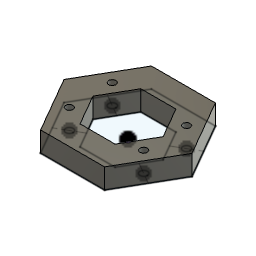
BrakeDiskSpacer (Autodesk Fusion 360 design; units mm, degrees)
Autodesk Fusion 360 part; units mm, degrees
sketch "Spacer" plane through (0, 0, 0) normal (0, 1, 0) x (1, 0, 0)
  line L0 (7.0148, 12.15) -> (-7.0148, 12.15)
  line L1 (-7.0148, 12.15) -> (-14.0296, 0)
  line L2 (-14.0296, 0) -> (-7.0148, -12.15)
  line L3 (-7.0148, -12.15) -> (7.0148, -12.15)
  line L4 (7.0148, -12.15) -> (14.0296, 0)
  line L5 (14.0296, 0) -> (7.0148, 12.15)
  line L6 (-12.7883, 22.15) -> (-25.5766, 0)
  line L7 (-25.5766, 0) -> (-12.7883, -22.15)
  line L8 (-12.7883, -22.15) -> (12.7883, -22.15)
  line L9 (12.7883, -22.15) -> (25.5766, 0)
  line L10 (25.5766, 0) -> (12.7883, 22.15)
  line L11 (12.7883, 22.15) -> (-12.7883, 22.15)
  line L12 (-19.1825, 11.075) -> (-10.5222, 6.075) construction
  line L13 (10.5222, 6.075) -> (19.1825, 11.075) construction
  line L14 (10.5222, -6.075) -> (19.1825, -11.075) construction
  line L15 (-10.5222, -6.075) -> (-19.1825, -11.075) construction
  circle A0 centre (-14.8523, 8.575) radius 1.45
  circle A1 centre (14.8523, 8.575) radius 1.45
  circle A2 centre (14.8523, -8.575) radius 1.45
  circle A3 centre (-14.8523, -8.575) radius 1.45
  dimension "d2" = 12.15
  dimension "d3" = 10
  dimension "d5" = 2.9
  dimension "d6" = 2.9
  dimension "d7" = 2.9
  dimension "d8" = 2.9
  constraint horizontal L8
  constraint horizontal L3
  constraint coincident L6 L12.start
  constraint coincident L1 L12.end
  constraint perpendicular L1 L12
  constraint midpoint L5 L13.start
  constraint midpoint L10 L13.end
  constraint midpoint L4 L14.start
  constraint coincident L9 L14.end
  constraint coincident L2 L15.start
  constraint coincident L7 L15.end
  constraint perpendicular L7 L15
  constraint midpoint L2 L15.start
  constraint midpoint L9 L14.end
  constraint midpoint L6 L12.start
  constraint midpoint L12 A0.centre
  constraint midpoint L13 A1.centre
  constraint coincident L14 A2.centre
  constraint coincident L15 A3.centre
  constraint midpoint L14 A2.centre
  constraint midpoint L15 A3.centre
  measures "d2" distance of origin L5
  measures "d5" diameter of A0
  measures "d6" diameter of A1
  measures "d7" diameter of A2
  measures "d8" diameter of A3
extrude "Extrude1" add sketch "Spacer" along normal blind 8
sketch "Lock nut hole" plane through (0, 0, 0) normal (0, 1, 0) x (1, 0, 0)
  line L0 (-11.6192, 8.575) -> (-13.2358, 11.375)
  line L1 (-13.2358, 11.375) -> (-16.4689, 11.375)
  line L2 (-16.4689, 11.375) -> (-18.0855, 8.575)
  line L3 (-18.0855, 8.575) -> (-16.4689, 5.775)
  line L4 (-16.4689, 5.775) -> (-13.2358, 5.775)
  line L5 (-13.2358, 5.775) -> (-11.6192, 8.575)
  line L6 (16.4689, 11.375) -> (13.2358, 11.375)
  line L7 (13.2358, 11.375) -> (11.6192, 8.575)
  line L8 (11.6192, 8.575) -> (13.2358, 5.775)
  line L9 (13.2358, 5.775) -> (16.4689, 5.775)
  line L10 (16.4689, 5.775) -> (18.0855, 8.575)
  line L11 (18.0855, 8.575) -> (16.4689, 11.375)
  line L12 (16.4689, -5.775) -> (13.2358, -5.775)
  line L13 (13.2358, -5.775) -> (11.6192, -8.575)
  line L14 (11.6192, -8.575) -> (13.2358, -11.375)
  line L15 (13.2358, -11.375) -> (16.4689, -11.375)
  line L16 (16.4689, -11.375) -> (18.0855, -8.575)
  line L17 (18.0855, -8.575) -> (16.4689, -5.775)
  line L18 (-11.6192, -8.575) -> (-13.2358, -5.775)
  line L19 (-13.2358, -5.775) -> (-16.4689, -5.775)
  line L20 (-16.4689, -5.775) -> (-18.0855, -8.575)
  line L21 (-18.0855, -8.575) -> (-16.4689, -11.375)
  line L22 (-16.4689, -11.375) -> (-13.2358, -11.375)
  line L23 (-13.2358, -11.375) -> (-11.6192, -8.575)
  line L24 (-19.1825, 11.075) -> (-10.5222, 6.075)
  line L25 (10.5222, 6.075) -> (19.1825, 11.075)
  line L26 (-10.5222, -6.075) -> (-19.1825, -11.075)
  line L27 (10.5222, -6.075) -> (19.1825, -11.075)
  point P0 (-14.8523, 8.575)
  point P1 (14.8523, 8.575)
  point P2 (14.8523, -8.575)
  point P3 (-14.8523, -8.575)
  dimension "d11" = 2.8
  dimension "d12" = 2.8
  dimension "d13" = 2.8
  dimension "d14" = 2.8
  constraint horizontal L4
  constraint horizontal L22
  constraint horizontal L15
  constraint horizontal L9
  constraint midpoint P0 L24
  constraint midpoint P1 L25
  constraint midpoint P3 L26
  constraint midpoint P2 L27
  measures "d11" distance of P0 L5
  measures "d12" distance of P1 L11
  measures "d13" distance of P2 L17
  measures "d14" distance of P3 L23
extrude "Extrude2" [suppressed]
move_body "Move1" [suppressed]
